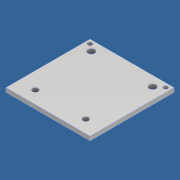
# Autodesk Inventor part: PlaqueGuideBlocLame
Saved by Autodesk Inventor 2018 (Build 220112000, 112)
## iProperties
Created: 2022-03-10
Part Number: PlaqueGuideBlocLame
Material: Aluminum 6061
Document SubType Name: Modeling
Designer: Nathann
Density: 2.7 g/cm^3
Appearance: Aluminum - Flat
Mass: 132.189 g
Surface Area: 221.993 cm^2
Volume: 48.9589 cm^3
Author: Nathann
Autodesk Inventor part; units mm, degrees
ref_plane "YZ Plane" through (0, 0, 0) normal (1, 0, 0) x (0, 1, 0)
ref_plane "XZ Plane" through (0, 0, 0) normal (0, 1, 0) x (-1, 0, 0)
ref_plane "XY Plane" through (0, 0, 0) normal (0, 0, 1) x (1, 0, 0)
sketch "Sketch1" plane through (0, 0, 0) normal (0, 0, 1) x (1, 0, 0)
  line L0 (0, 0) -> (-100, 0)
  line L1 (-100, 0) -> (-100, 100)
  line L2 (-100, 100) -> (0, 100)
  line L3 (0, 100) -> (0, 0)
  dimension "d0" = 100
  dimension "d1" = 100
  constraints: 8 end point, 2 parallel, 1 horizontal, 1 perpendicular
  measures "d0" distance of L2.end L0.start
  measures "d1" distance of L1.end L2.end
extrude "Extrusion1" add sketch "Sketch1" along normal blind 5
sketch "Sketch11" plane through (-80, 15, 0) normal (0, 0, -1) x (-1, 0, 0)
  circle A0 centre (0, 0) radius 3.3
  circle A1 centre (-30, 0) radius 5 projected
  circle A2 centre (-30, 0) radius 3
  circle A3 centre (-60, 0) radius 5 projected
  circle A4 centre (-60, 0) radius 3.3
  point P0 (-80, -15)
  dimension "d101" = 6.6
  dimension "d102" = 6
  dimension "d103" = 6.6
  constraints: 3 centre point, 2 coincident
  measures "d101" diameter of A0
  measures "d102" diameter of A2
  measures "d103" diameter of A4
extrude "Extrusion11" cut sketch "Sketch11" along normal through all both and the other way through all contours A0 | A4
sketch "Sketch7" plane through (0, 0, 0) normal (0, 0, -1) x (-1, 0, 0)
  line L0 (100, 25) -> (0, 25)
  line L1 (100, 56.2495) -> (100, 25)
  line L2 (100, 100) -> (0, 100)
  line L3 (0, 0) -> (100, 0) projected
  circle A0 centre (86.5, 88) radius 4
  circle A1 centre (86.5, 88) radius 1.65
  line L4 (50, 100) -> (50, 0)
  line L5 (100, 0) -> (0, 0) projected
  line L6 (0, 100) -> (0, 100)
  line L7 (0, 100) -> (0, 98.5)
  circle A2 centre (95, 95) radius 2.5
  line L8 (100, 0) -> (100, 100) projected
  line L9 (0, 0) -> (100, 0) projected
  line L10 (100, 0) -> (100, 100) projected
  line L11 (100, 100) -> (0, 100) projected
  line L12 (0, 100) -> (0, 0) projected
  circle A3 centre (13.5, 88) radius 4
  circle A4 centre (13.5, 88) radius 1.65
  circle A5 centre (5, 95) radius 2.5
  point P0 (95.4835, 97.4528)
  point P1 (95.4244, 97.4637)
  point P2 (0, 100)
  point P3 (0, 100)
  point P4 (4.5165, 97.4528)
  point P5 (4.5756, 97.4637)
  point P6 (0, 100)
  dimension "d72" = 25
  dimension "d77" = 8
  dimension "d78" = 3.3
  dimension "d88" = 5
  dimension "d111" = 5
  dimension "d112" = 8.5
  dimension "d121" = 7
  dimension "d122" = 5
  constraints: 12 end point, 8 symmetric about line, 6 centre point, 4 point on circle, 2 coincident, 2 horizontal, 2 midpoint, 3 other
  measures "d72" distance between parallel lines of L0 L3
  measures "d77" diameter of A0
  measures "d78" diameter of A1
  measures "d88" diameter of A2
  measures "d111" distance from line of L8 A2.centre
  measures "d112" horizontal distance of A2.centre A0.centre
  measures "d121" vertical distance of A0.centre A2.centre
  measures "d122" distance from line of L2 A2.centre
extrude "Extrusion13" cut sketch "Sketch7" against normal blind 10 contours A0 | A1 | A2 | A3 | A4 | A5
sketch "Sketch13" plane through (0, 0, 5) normal (0, 0, 1) x (1, 0, 0)
  line L0 (-10, 25) -> (-90, 25) construction
  line L1 (-90, 25) -> (-90, 85) construction
  line L2 (-90, 85) -> (-10, 85) construction
  line L3 (-10, 85) -> (-10, 25) construction
  line L4 (0, 0) -> (0, 100) projected
  line L5 (-100, 100) -> (-100, 0) projected
  line L6 (-100, 0) -> (0, 0) projected
  dimension "d123" = 10
  dimension "d124" = 80
  dimension "d125" = 60
  dimension "d126" = 100
  dimension "d127" = 25
  constraints: 2 other
  measures "d123" distance between parallel lines of L4 L3
  measures "d124" distance between parallel lines of L3 L1
  measures "d125" distance between parallel lines of L0 L2
  measures "d126" distance between parallel lines of L5 L4
  measures "d127" distance between parallel lines of L6 L0
equation "\"d103\" = d101"
equation "\"d88\" = d86"
equation "\"d123\" = -0.5 * d124 + 0.5 * d126"
equation "\"d86\" = 5"
body "Solid1"
